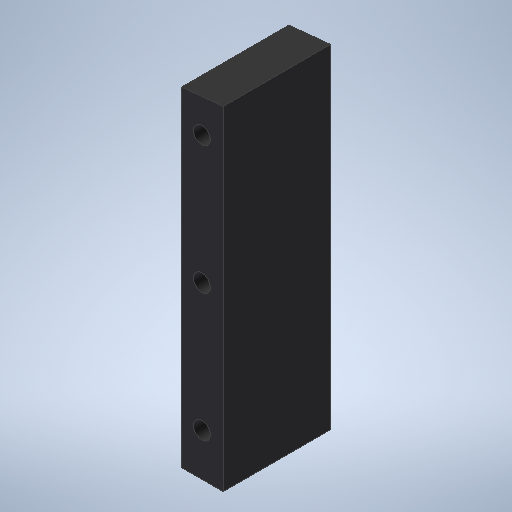
# Autodesk Inventor part: ReleaseMec2.0SideWall
Saved by Autodesk Inventor 2025 (Build 290162000, 162)
## iProperties
Created: 2025-11-13
Part Number: ReleaseMec2.0SideWall
Material: Generic
Document SubType Name: Modeling
Designer: ruven
Density: 1 g/cm^3
Appearance: Default
Author: ruven
Autodesk Inventor part; units mm, degrees
ref_plane "YZ Plane" through (0, 0, 0) normal (1, 0, 0) x (0, 1, 0)
ref_plane "XZ Plane" through (0, 0, 0) normal (0, 1, 0) x (-1, 0, 0)
ref_plane "XY Plane" through (0, 0, 0) normal (0, 0, 1) x (1, 0, 0)
sketch "Sketch1" plane through (0, 0, 0) normal (0, 0, 1) x (1, 0, 0)
  line L0 (4.9, 12.6) -> (-4.9, 12.6)
  line L1 (-4.9, 12.6) -> (-4.9, -12.6)
  line L2 (-4.9, -12.6) -> (4.9, -12.6)
  line L3 (4.9, -12.6) -> (4.9, 12.6)
  line L4 (4.9, 12.6) -> (-4.9, -12.6) construction
  line L5 (-4.9, 12.6) -> (4.9, -12.6) construction
  point P0 (0, 0)
  dimension "d0" = 25.2
  dimension "d1" = 9.8
  constraints: 12 end point, 2 midpoint, 2 parallel, 1 horizontal, 1 perpendicular
  measures "d0" distance of L0.end L1.end
  measures "d1" distance of L0.start L0.end
extrude "Extrusion1" add sketch "Sketch1" along normal blind 80
sketch "Sketch2" plane through (-4.9, 12.6, 0) normal (0, 1, 0) x (1, 0, 0)
  circle A0 centre (4.8, -70) radius 2
  circle A1 centre (4.8, -40) radius 2
  circle A2 centre (4.8, -10) radius 2
  line L0 (9.8, -80) -> (0, -80) projected
  line L1 (9.8, 0) -> (0, 0) projected
  line L2 (9.8, 0) -> (9.8, -80) projected
  point P0 (4.9, 0)
  point P1 (9.8, -40)
  dimension "d4" = 4
  dimension "d5" = 4
  dimension "d6" = 4
  dimension "d7" = 10
  dimension "d8" = 10
  dimension "d9" = 40
  dimension "d10" = 5
  dimension "d11" = 5
  dimension "d12" = 5
  constraints: 3 centre point, 1 midpoint
  measures "d4" diameter of A0
  measures "d5" diameter of A1
  measures "d6" diameter of A2
  measures "d7" distance from line of L0 A0.centre
  measures "d8" distance from line of L1 A2.centre
  measures "d9" distance from line of L0 A1.centre
  measures "d10" distance from line of L2 A0.centre
  measures "d11" distance of point (9.8, -40) A1.centre
  measures "d12" distance from line of L2 A2.centre
extrude "Extrusion2" cut sketch "Sketch2" against normal blind 80
sketch "Sketch3" plane through (-4.9, -12.6, 0) normal (0, -1, 0) x (1, 0, 0)
  arc A0 (48.1, 80) -> (-9.1978, 76.2369) centre (48.1, -358.1) ccw
  line L0 (0, 80) -> (9.8, 80) projected
  line L1 (0, 0) -> (0, 80) projected
  line L2 (0, 80) -> (48.1, 80)
  line L3 (-9.1978, 76.2369) -> (-9.1978, 80)
  line L4 (-9.1978, 80) -> (0, 80)
  point P0 (4.9, 0)
  point P1 (4.9, 80)
  dimension "d15" = 876.2
  dimension "d17" = 48.1
  dimension "d18" = 438.1
  constraints: 6 end point, 2 point on circle, 1 centre point, 1 collinear, 1 horizontal, 1 midpoint, 1 vertical
  measures "d15" diameter of A0
  measures "d17" distance from line of A0.centre L1
  measures "d18" distance from line of A0.centre L2
extrude "Extrusion3" cut sketch "Sketch3" against normal through all
body "Solid1"
